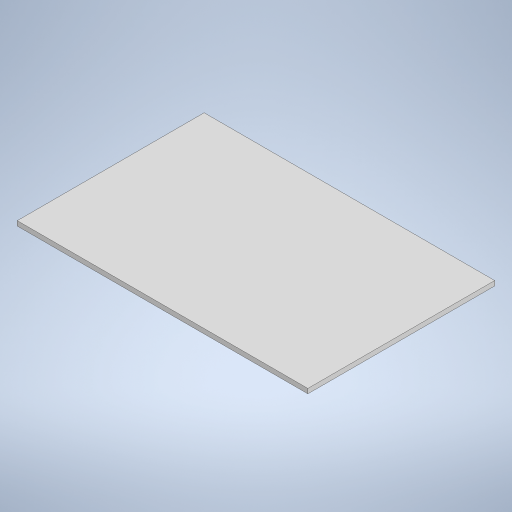
# Autodesk Inventor part: Lid
Saved by Autodesk Inventor 2023 (Build 270158000, 158)
## iProperties
Created: 2023-02-08
Part Number: Lid
Material: Generic
Document SubType Name: Modeling
Designer: Ahmed Nazir
Density: 1 g/cm^3
Appearance: Default
Author: Ahmed Nazir
Autodesk Inventor part; units mm, degrees
ref_plane "YZ Plane" through (0, 0, 0) normal (1, 0, 0) x (0, 1, 0)
ref_plane "XZ Plane" through (0, 0, 0) normal (0, 1, 0) x (-1, 0, 0)
sketch "Sketch1" plane through (0, 0, 0) normal (0, 1, 0) x (-1, 0, 0)
  line L0 (90, -113.6) -> (-90, -113.6)
  line L1 (-90, -113.6) -> (-90, 0)
  line L2 (-90, 0) -> (90, 0)
  line L3 (90, 0) -> (90, -113.6)
  line L4 (-93, -116.6) -> (93, -116.6)
  line L5 (93, -116.6) -> (93, 3)
  line L6 (93, 3) -> (-93, 3)
  line L7 (-93, 3) -> (-93, -116.6)
  point P0 (0, 0)
  point P1 (0, 0)
  dimension "d0" = 180
  dimension "d1" = 113.6
  dimension "d2" = 3
  constraints: 16 end point, 4 parallel, 2 perpendicular, 1 coincident, 1 horizontal, 1 midpoint, 3 other
  measures "d0" distance of L1.end L2.end
  measures "d1" distance of L0.end L1.end
  measures "d2" distance between parallel lines of L0 L4
extrude "Extrusion1" add sketch "Sketch1" along normal blind 3 contours L0 L1 L2 L3 | L7 L6 L5 L4
extrude "Extrusion2" add sketch "Sketch1" against normal blind 3 contours L0 L1 L2 L3
ref_plane "Work Plane1" through (-93, 0, -56.8) normal (0, 0, 1) x (1, 0, 0)
sketch "Sketch2" plane through (-93, 0, -56.8) normal (0, 0, 1) x (1, 0, 0)
  line L0 (0, 3) -> (186, 3) projected
  line L1 (159.34, 3) -> (146.166, 3)
  line L2 (146.166, 3) -> (142.9018, 10)
  line L3 (142.9018, 10) -> (162.6042, 10)
  line L4 (162.6042, 10) -> (159.34, 3)
  line L5 (119.506, 3) -> (106.332, 3)
  line L6 (106.332, 3) -> (103.0678, 10)
  line L7 (103.0678, 10) -> (122.7702, 10)
  line L8 (122.7702, 10) -> (119.506, 3)
  line L9 (93, 3) -> (93, -12.5812) construction
  line L10 (26.66, 3) -> (39.834, 3)
  line L11 (39.834, 3) -> (43.0982, 10)
  line L12 (43.0982, 10) -> (23.3958, 10)
  line L13 (23.3958, 10) -> (26.66, 3)
  line L14 (66.494, 3) -> (79.668, 3)
  line L15 (79.668, 3) -> (82.9322, 10)
  line L16 (82.9322, 10) -> (63.2298, 10)
  line L17 (63.2298, 10) -> (66.494, 3)
  point P0 (93, 0)
  point P1 (26.66, 3)
  point P2 (39.834, 3)
  point P3 (66.494, 3)
  point P4 (79.668, 3)
  dimension "d7" = 13.174
  dimension "d8" = 13.174
  dimension "d9" = 65
  dimension "d10" = 65
  dimension "d11" = 7
  dimension "d12" = 26.66
  dimension "d13" = 26.66
  constraints: 34 end point, 8 symmetric about line, 4 point on line, 3 equal length, 2 parallel, 1 midpoint, 1 vertical
  measures "d7" distance of L1.start L1.end
  measures "d8" distance of L5.start L5.end
  measures "d9" angle of L2 L0
  measures "d10" angle of L0 L4
  measures "d11" distance between parallel lines of L0 L3
  measures "d12" distance of L0.end L1.start
  measures "d13" distance of L5.start L1.end
extrude "Extrusion3" [suppressed]
sketch "Sketch3" plane through (0, -3, 0) normal (0, -1, 0) x (1, 0, 0)
  line L0 (-87, -3) -> (87, -3)
  line L1 (87, -3) -> (87, -110.6)
  line L2 (87, -110.6) -> (-87, -110.6)
  line L3 (-87, -110.6) -> (-87, -3)
  line L4 (90, 0) -> (-90, 0) projected
  line L5 (-90, 0) -> (-90, -113.6) projected
  line L6 (-90, -113.6) -> (90, -113.6) projected
  line L7 (90, -113.6) -> (90, 0) projected
  point P0 (0, 0)
  dimension "d16" = 3
  dimension "d17" = 3
  dimension "d18" = 3
  dimension "d19" = 3
  constraints: 8 end point, 2 parallel, 1 horizontal, 1 perpendicular
  measures "d16" distance between parallel lines of L4 L0
  measures "d17" distance between parallel lines of L5 L3
  measures "d18" distance between parallel lines of L6 L2
  measures "d19" distance between parallel lines of L7 L1
extrude "Extrusion4" cut sketch "Sketch3" against normal blind 3 contours L0 L1 L2 L3
body "Solid1"
